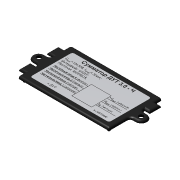
# Autodesk Inventor part: крышка Ч_А
Saved by Autodesk Inventor 2012 (Build 160160000, 160)
## iProperties
Created: 2009-09-07
Part Number: крышка Ч_А
Material: По умолчанию
Document SubType Name: Обычные детали
Designer: toma
Density: 1 g/cm^3
Mass: 4.00244 g
Surface Area: 57.6307 cm^2
Volume: 4.00244 cm^3
Sheet Metal Rule: По умолчанию_мм
Author: toma
Autodesk Inventor part; units mm, degrees
ref_plane "YZ Plane" through (0, 0, 0) normal (1, 0, 0) x (0, 1, 0)
ref_plane "XZ Plane" through (0, 0, 0) normal (0, 1, 0) x (-1, 0, 0)
ref_plane "XY Plane" through (0, 0, 0) normal (0, 0, 1) x (1, 0, 0)
sketch "Эскиз1" plane through (0, 0, 0) normal (0, 0, 1) x (1, 0, 0)
  line L0 (29, 24) -> (-36, 24)
  line L1 (-36, 24) -> (-36, 19)
  line L2 (-36, 19) -> (-40, 19)
  line L3 (-40, 19) -> (-40, 11)
  line L4 (-40, 11) -> (-36, 11)
  line L5 (-36, 11) -> (-36, 11)
  line L6 (-38, 9) -> (-40, 9)
  line L7 (-44, 5) -> (-44, 5)
  line L8 (-40, 1) -> (-38, 1)
  line L9 (-36, -1) -> (-36, -1)
  line L10 (-36, -1) -> (-40, -1)
  line L11 (-40, -1) -> (-40, -9)
  line L12 (-40, -9) -> (-36, -9)
  line L13 (-36, -9) -> (-36, -14)
  line L14 (-36, -14) -> (29, -14)
  line L15 (29, -14) -> (29, -1)
  line L16 (31, 1) -> (33, 1)
  line L17 (37, 5) -> (37, 5)
  line L18 (33, 9) -> (31.3808, 9)
  line L19 (29.3808, 11) -> (29.3808, 11)
  line L20 (29.3808, 11) -> (33, 11)
  line L21 (33, 11) -> (33, 11)
  line L22 (33, 11) -> (33, 19)
  line L23 (33, 19) -> (29, 19)
  line L24 (29, 19) -> (29, 24)
  arc A0 (29.3808, 11) -> (31.3808, 9) centre (31.3808, 11) ccw
  arc A1 (-38, 9) -> (-36, 11) centre (-38, 11) ccw
  arc A2 (-36, -1) -> (-38, 1) centre (-38, -1) ccw
  arc A3 (31, 1) -> (29, -1) centre (31, -1) ccw
  arc A4 (-40, 9) -> (-44, 5) centre (-40, 5) ccw
  arc A5 (-44, 5) -> (-40, 1) centre (-40, 5) ccw
  arc A6 (37, 5) -> (33, 9) centre (33, 5) ccw
  arc A7 (33, 1) -> (37, 5) centre (33, 5) ccw
  point P0 (-36, 9)
  point P1 (-44, 9)
  point P2 (-44, 1)
  point P3 (-36, 1)
  dimension "d0" = 65
  dimension "d1" = 65
  dimension "d2" = 4
  dimension "d3" = 38
  dimension "d4" = 8
  dimension "d5" = 2
  dimension "d6" = 2
  dimension "d7" = 8
  dimension "d8" = 8
  dimension "d11" = 4
  dimension "d12" = 8
  dimension "d13" = 2
  dimension "d14" = 8
  dimension "d16" = 8
  dimension "d17" = 2
  dimension "d18" = 8
  dimension "d19" = 4
  dimension "d20" = 2
  dimension "d21" = 4
  dimension "d68" = 19
  dimension "d69" = 19
  constraints: 50 end point, 18 parallel, 16 point on circle, 16 tangent, 11 point on line, 8 centre point, 5 equal radius, 3 collinear, 3 perpendicular, 1 horizontal
  measures "d0" distance of L0.start L0.end
  measures "d1" distance of L13.end L14.end
  measures "d2" distance of L22.end L23.end
  measures "d3" distance between parallel lines of L14 L0
  measures "d4" distance between parallel lines of L20 L23
  measures "d5" distance between parallel lines of L18 L20
  measures "d6" radius of A0
  measures "d7" distance between parallel lines of L16 L18
  measures "d8" distance between parallel lines of L17 L15
  measures "d11" distance of L1.end L2.end
  measures "d12" distance of L2.end L3.end
  measures "d13" distance of L4.end point (-36, 9)
  measures "d14" distance of point (-44, 9) point (-44, 1)
  measures "d16" distance of point (-44, 1) point (-36, 1)
  measures "d17" distance of point (-36, 1) L9.end
  measures "d18" distance of L10.end L11.end
  measures "d19" distance of L11.end L12.end
  measures "d20" radius of A1
  measures "d21" radius of A4
  measures "d68" distance from line of A5.centre L0
  measures "d69" distance from line of L0 A7.centre
extrude "Выдавливание1" add sketch "Эскиз1" along normal blind 1.5
sketch "Эскиз2" plane through (0, 0, 1.5) normal (0, 0, 1) x (1, 0, 0)
  circle A0 centre (-39.8, 5) radius 1.6
  circle A1 centre (32.8, 5) radius 1.6
  dimension "d53" = 3.2
  dimension "d54" = 3.2
  dimension "d55" = 72.6
  constraints: 2 centre point
  measures "d53" diameter of A0
  measures "d54" diameter of A1
  measures "d55" distance of A1.centre A0.centre
extrude "Выдавливание2" cut sketch "Эскиз2" against normal blind 10
sketch "Эскиз3" plane through (0, 0, 0) normal (0, 0, -1) x (-1, 0, 0)
  line L0 (30.75, 23) -> (-23.75, 23)
  line L1 (-24, 22.75) -> (-24, 21.75)
  line L2 (-23.75, 21.5) -> (30.75, 21.5)
  line L3 (31, 21.75) -> (31, 22.75)
  line L4 (-23.75, -11.5) -> (30.75, -11.5)
  line L5 (31, -11.75) -> (31, -12.75)
  line L6 (30.75, -13) -> (-23.75, -13)
  line L7 (-24, -12.75) -> (-24, -11.75)
  line L8 (-28.25, 11) -> (-27.75, 11)
  line L9 (-27.5, 10.75) -> (-27.5, -0.75)
  line L10 (-27.75, -1) -> (-28.25, -1)
  line L11 (-28.5, -0.75) -> (-28.5, 10.75)
  line L12 (34.75, 11) -> (35.25, 11)
  line L13 (35.5, 10.75) -> (35.5, -0.75)
  line L14 (35.25, -1) -> (34.75, -1)
  line L15 (34.5, -0.75) -> (34.5, 10.75)
  line L16 (3.5, -14) -> (3.5, 26) construction
  arc A0 (-27.5, 10.75) -> (-27.75, 11) centre (-27.75, 10.75) ccw
  arc A1 (-28.25, 11) -> (-28.5, 10.75) centre (-28.25, 10.75) ccw
  arc A2 (-27.75, -1) -> (-27.5, -0.75) centre (-27.75, -0.75) ccw
  arc A3 (-28.5, -0.75) -> (-28.25, -1) centre (-28.25, -0.75) ccw
  arc A4 (35.5, 10.75) -> (35.25, 11) centre (35.25, 10.75) ccw
  arc A5 (34.75, 11) -> (34.5, 10.75) centre (34.75, 10.75) ccw
  arc A6 (35.25, -1) -> (35.5, -0.75) centre (35.25, -0.75) ccw
  arc A7 (34.5, -0.75) -> (34.75, -1) centre (34.75, -0.75) ccw
  arc A8 (30.75, 21.5) -> (31, 21.75) centre (30.75, 21.75) ccw
  arc A9 (31, 22.75) -> (30.75, 23) centre (30.75, 22.75) ccw
  arc A10 (-23.75, 23) -> (-24, 22.75) centre (-23.75, 22.75) ccw
  arc A11 (-24, 21.75) -> (-23.75, 21.5) centre (-23.75, 21.75) ccw
  arc A12 (-23.75, -11.5) -> (-24, -11.75) centre (-23.75, -11.75) ccw
  arc A13 (-24, -12.75) -> (-23.75, -13) centre (-23.75, -12.75) ccw
  arc A14 (-23.75, -11.5) -> (-24, -11.75) centre (-23.75, -11.75) ccw
  arc A15 (30.75, -13) -> (31, -12.75) centre (30.75, -12.75) ccw
  arc A16 (31, -11.75) -> (30.75, -11.5) centre (30.75, -11.75) ccw
  point P0 (31, 23)
  point P1 (-24, 23)
  point P2 (-24, 21.5)
  point P3 (31, 21.5)
  point P4 (-24, -11.5)
  point P5 (31, -11.5)
  point P6 (31, -13)
  point P7 (-24, -13)
  point P8 (-28.5, 11)
  point P9 (-27.5, 11)
  point P10 (-27.5, -1)
  point P11 (-28.5, -1)
  point P12 (34.5, 11)
  point P13 (35.5, 11)
  point P14 (35.5, -1)
  point P15 (34.5, -1)
  dimension "d30" = 55
  dimension "d32" = 55
  dimension "d35" = 1.5
  dimension "d37" = 1.5
  dimension "d38" = 12
  dimension "d39" = 12
  dimension "d40" = 1
  dimension "d41" = 1
  dimension "d49" = 27.5
  dimension "d50" = 27.5
  dimension "d58" = 0.25
  dimension "d59" = 0.25
  constraints: 34 end point, 34 point on circle, 34 point on line, 34 tangent, 17 centre point, 15 equal radius, 8 perpendicular, 7 parallel
  measures "d30" distance of point (31, 23) point (-24, 23)
  measures "d32" distance of point (31, -13) point (-24, -13)
  measures "d35" distance of point (-24, 23) point (-24, 21.5)
  measures "d37" distance between parallel lines of L4 L6
  measures "d38" distance of point (-28.5, -1) point (-28.5, 11)
  measures "d39" distance of point (35.5, 11) point (35.5, -1)
  measures "d40" distance of point (35.5, -1) point (34.5, -1)
  measures "d41" distance of point (-27.5, -1) point (-28.5, -1)
  measures "d49" distance between parallel lines of L5 L16
  measures "d50" distance between parallel lines of L3 L16
  measures "d58" radius of A0
  measures "d59" radius of A4
extrude "Выдавливание3" add sketch "Эскиз3" along normal blind 0.5
sketch "Эскиз5" plane through (0, 0, 0) normal (0, 0, -1) x (-1, 0, 0)
  circle A0 centre (-32.8, 5) radius 1.6 projected
  circle A1 centre (39.8, 5) radius 1.6 projected
  circle A2 centre (-26.5, 21.5) radius 1
  circle A3 centre (33.5, 21.5) radius 1
  circle A4 centre (33.5, -11.5) radius 1
  circle A5 centre (-26.5, -11.5) radius 1
  dimension "d60" = 2
  dimension "d61" = 2
  dimension "d62" = 2
  dimension "d63" = 2
  dimension "d65" = 16.5
  dimension "d66" = 16.5
  dimension "d67" = 16.5
  constraints: 4 centre point
  measures "d60" diameter of A2
  measures "d61" diameter of A3
  measures "d62" diameter of A4
  measures "d63" diameter of A5
  measures "d65" vertical distance of A3.centre A1.centre
  measures "d66" vertical distance of A5.centre A0.centre
  measures "d67" vertical distance of A1.centre A4.centre
extrude "Выдавливание4" add sketch "Эскиз5" along normal blind 2.5 contours A2 | A3 | A4 | A5
fillet "Сопряжение3" radius 1 4 edges at (27.5, 21.5, -2.5) (27.5, -11.5, -2.5) (-32.5, -11.5, -2.5) (-32.5, 21.5, -2.5)
fillet "Сопряжение4" radius 1.5 4 edges at (-36, -14, 0.75) (29, -14, 0.75) (29, 24, 0.75) (-36, 24, 0.75)
fillet "Сопряжение5" radius 1.5 29 edges at (-3.5, -14, 1.5) (-35.5607, -13.5607, 1.5) (-36, -10.75, 1.5) (28.5607, -13.5607, 1.5) (29, -6.75, 1.5) (29.5858, 0.4142, 1.5) (32, 1, 1.5) (37, 5, 1.5) (32.1904, 9, 1.5) (29.9666, 9.5858, 1.5) (31.1904, 11, 1.5) (33, 15, 1.5) (31, 19, 1.5) (29, 20.75, 1.5) (28.5607, 23.5607, 1.5) (-3.5, 24, 1.5) (-35.5607, 23.5607, 1.5) (-36, 20.75, 1.5) (-38, 19, 1.5) (-38, 11, 1.5) (-40, 15, 1.5) (-36.5858, 9.5858, 1.5) (-39, 9, 1.5) (-44, 5, 1.5) (-39, 1, 1.5) (-36.5858, 0.4142, 1.5) (-38, -1, 1.5) (-40, -5, 1.5) (-38, -9, 1.5)
sketch "Эскиз9" plane through (0, 0, 1.5) normal (0, 0, 1) x (1, 0, 0)
  line L0 (-31, 20) -> (25.1976, 20) construction
  line L1 (25.1976, 20) -> (25.1976, -10.2049) construction
  line L2 (25.1976, -10.2049) -> (-31, -10.2049) construction
  line L3 (-31, -10.2049) -> (-31, 20) construction
  point P0 (0, 0)
  constraints: 2 other
decal "Маркировка4"
equation "\"Радиус_гибки\" = Толщина"
equation "\"Ширина_просечки\" = Толщина"
equation "\"Глубина_просечки\" = 0.5 * Толщина"
equation "\"Размер_высечки\" = 4 * Толщина"
equation "\"Мин_остаток\" = 2 * Толщина"
equation "\"Радиус_перехода\" = Радиус_гибки"
equation "\"Радиус_Якоби\" = Радиус_гибки"
equation "\"Размер_зазора\" = Толщина"
equation "\"Толщина\" = 0.5"
